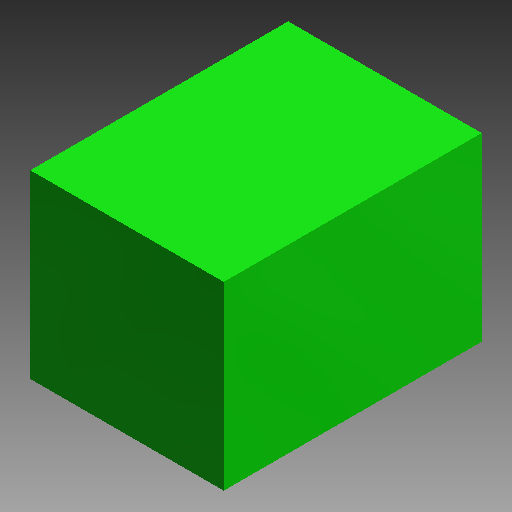
# Autodesk Inventor part: 1571610-2
Saved by Autodesk Inventor 2018.2 (Build 222227000, 227)
## iProperties
Part Number: 1571610-2
Material: Generic
Document SubType Name: Modeling
Designer: autocad
Appearance: B3F-31XX, 1571610-2
Author: autocad
Autodesk Inventor part; units mm, degrees
ref_plane "YZ Plane" through (0, 0, 0) normal (1, 0, 0) x (0, 1, 0)
ref_plane "XZ Plane" through (0, 0, 0) normal (0, 1, 0) x (-1, 0, 0)
ref_plane "XY Plane" through (0, 0, 0) normal (0, 0, 1) x (1, 0, 0)
sketch "B3F-31XX, 1571610-2_309" plane through (0, 0, 0) normal (0, 0, 1) x (1, 0, 0)
  line L0 (4.2, 2.77) -> (4.2, -5.08)
  line L1 (4.2, -5.08) -> (-4.2, -5.08)
  line L2 (-4.2, -5.08) -> (-4.2, 2.77)
  line L3 (-4.2, 2.77) -> (4.2, 2.77)
  constraints: 8 end point
extrude "Extrusion1" add sketch "B3F-31XX, 1571610-2_309" along normal blind 11.2
body "Solid1"
